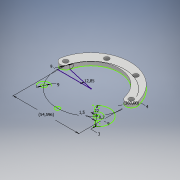
# Autodesk Inventor part: fin entraineur mod
Saved by Autodesk Inventor 2018.1 (Build 221171000, 171)
## iProperties
Created: 2022-06-22
Part Number: fin entraineur mod
Material: Generic
Document SubType Name: Modeling
Designer: mouta
Density: 1 g/cm^3
Appearance: Default
Author: mouta
Autodesk Inventor part; units mm, degrees
ref_plane "YZ Plane" through (0, 0, 0) normal (1, 0, 0) x (0, 1, 0)
ref_plane "XZ Plane" through (0, 0, 0) normal (0, 1, 0) x (-1, 0, 0)
ref_plane "XY Plane" through (0, 0, 0) normal (0, 0, 1) x (1, 0, 0)
sketch "Sketch1" plane through (0, 0, 0) normal (0, 0, 1) x (1, 0, 0)
  circle A0 centre (27.2972, 6.234) radius 2
  circle A1 centre (12.1456, 25.2286) radius 2
  circle A2 centre (-12.1519, 25.2256) radius 2
  circle A3 centre (-27.2988, 6.2272) radius 2
  circle A4 centre (-21.8891, -17.4604) radius 2
  circle A5 centre (0.0035, -28) radius 2
  circle A6 centre (21.8935, -17.455) radius 2
  arc A7 (-18.3712, -14.6543) -> (-25.407, -20.2666) centre (-21.8891, -17.4604) ccw
  arc A8 (-31.6861, 7.228) -> (-22.9115, 5.2264) centre (-27.2988, 6.2272) ccw
  line L0 (0, 0) -> (-27.2988, 6.2272)
  line L1 (0, 0) -> (-28.0096, 0)
  arc A9 (22.9102, 5.2321) -> (31.6843, 7.2359) centre (27.2972, 6.234) ccw
  arc A10 (25.412, -20.2603) -> (18.3749, -14.6497) centre (21.8935, -17.455) ccw
  arc A11 (18.3162, -14.7229) -> (18.3749, -14.6497) centre (0, 0) ccw
  arc A12 (22.9102, 5.2321) -> (-22.9115, 5.2264) centre (0, 0) ccw
  arc A13 (25.3999, -20.2755) -> (25.412, -20.2603) centre (0, 0) ccw
  arc A14 (31.6843, 7.2359) -> (-31.6861, 7.228) centre (0, 0) ccw
  arc A15 (31.3012, -23.1554) -> (15.9051, -8.2279) centre (21.8935, -17.455) ccw
  line L2 (21.8935, -17.455) -> (20.255, -16.308)
  line L3 (18.0457, -14.7615) -> (15.8179, -13.202)
  line L4 (21.8935, -17.455) -> (23.0905, -19.0572)
  line L5 (25.3705, -22.1091) -> (26.3321, -23.3962)
  arc A16 (25.3999, -20.2755) -> (25.3705, -22.1091) centre (26.5722, -21.2113) ccw
  arc A17 (26.3321, -23.3962) -> (31.3012, -23.1554) centre (28.7355, -21.6007) ccw
  arc A18 (15.9051, -8.2279) -> (15.8179, -13.202) centre (17.5383, -10.7444) ccw
  arc A19 (18.0457, -14.7615) -> (18.3162, -14.7229) centre (18.1604, -14.5976) ccw
  point P0 (28.477, -26.2673)
  point P1 (12.8819, -11.1468)
  point P2 (18.1984, -14.8684)
  point P3 (24.6644, -21.164)
  dimension "d2" = 4
  dimension "d5" = 360
  dimension "d7" = 9
  dimension "d8" = 9
  dimension "d11" = 12.85
  dimension "d12" = 54.596
  dimension "d13" = 9
  dimension "d14" = 22
  dimension "d15" = 1.5
  dimension "d16" = 3
  dimension "d17" = 0.2
  constraints: 34 point on circle, 20 centre point, 12 end point, 8 tangent, 7 coincident, 4 point on line, 1 equal radius, 1 horizontal, 15 other
  measures "d2" diameter of A0
  measures "d7" diameter of A7
  measures "d8" diameter of A8
  measures "d11" angle of L1 L0
  measures "d12" distance of A0.centre A3.centre
  measures "d13" diameter of A10
  measures "d14" diameter of A15
  measures "d15" radius of A16
  measures "d16" radius of A17
  measures "d17" radius of A19
extrude "Extrusion1" add sketch "Sketch1" along normal blind 3 contours A14 A9 A12 A8
body "Solid1"
